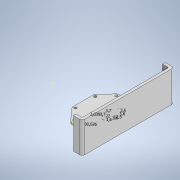
# Autodesk Inventor part: pare_choc_demo_reel
Saved by Autodesk Inventor 2020.4 (Build 244396000, 396)
## iProperties
Created: 2021-07-13
Part Number: pare_choc_demo_reel
Material: Generic
Document SubType Name: Modeling
Designer: Antonin Betaille
Density: 1 g/cm^3
Appearance: Default
Author: Antonin Betaille
Autodesk Inventor part; units mm, degrees
ref_plane "YZ Plane" through (0, 0, 0) normal (1, 0, 0) x (0, 1, 0)
ref_plane "XZ Plane" through (0, 0, 0) normal (0, 1, 0) x (-1, 0, 0)
ref_plane "XY Plane" through (0, 0, 0) normal (0, 0, 1) x (1, 0, 0)
sketch "Sketch1" plane through (0, 0, 0) normal (0, 1, 0) x (-1, 0, 0)
  line L0 (0, 34) -> (16, 16) construction
  line L1 (18.9896, 18.6575) -> (2.9896, 36.6575)
  arc A0 (2.9896, 36.6575) -> (0, 38) centre (0, 34) ccw
  arc A1 (20, 16) -> (18.9896, 18.6575) centre (16, 16) ccw
  line L2 (16, 16) -> (16, -16) construction
  line L3 (20, -16) -> (20, 16)
  line L4 (16, -16) -> (0, -34) construction
  line L5 (2.9896, -36.6575) -> (18.9896, -18.6575)
  line L6 (0, 34) -> (-44.6053, 34) construction
  line L7 (0, 38) -> (-53, 38)
  line L8 (0, -34) -> (-49, -34) construction
  line L9 (-53, -38) -> (0, -38)
  line L10 (-49, 30.0008) -> (-49, -29.9992) construction
  line L11 (-53, 38) -> (-53, -38)
  arc A2 (18.9896, -18.6575) -> (20, -16) centre (16, -16) ccw
  arc A3 (0, -38) -> (2.9896, -36.6575) centre (0, -34) ccw
  point P0 (0, 0)
  point P1 (8, 25)
  point P2 (16, 0)
  point P3 (8, -25)
  point P4 (-24.1053, 34)
  point P5 (-24.5, -34)
  point P6 (-49, 0.0008)
  dimension "d1" = 34
  dimension "d2" = 32
  dimension "d3" = 16
  dimension "d4" = 16
  dimension "d6" = 8
  dimension "d12" = 4
  dimension "d13" = 4
  dimension "d15" = 4
  dimension "d17" = 68
  dimension "d18" = 76
  dimension "d19" = 73
  dimension "d21" = 20
  dimension "d40" = 76
  dimension "d41" = 53
  constraints: 33 end point, 8 point on circle, 8 tangent, 5 midpoint, 4 centre point, 2 point on line
  measures "d1" distance of L0.start point (0, 0)
  measures "d2" distance of L2.end L0.end
  measures "d3" horizontal distance of L0.end L0.start
  measures "d4" horizontal distance of point (0, 0) L0.end
  measures "d6" diameter of A1
  measures "d12" radius of A3
  measures "d13" radius of A0
  measures "d15" radius of A2
  measures "d17" distance of L0.start L4.end
  measures "d18" distance between parallel lines of L9 L7
  measures "d19" distance between parallel lines of L11 L3
  measures "d21" distance from line of point (0, 0) L3
  measures "d40" distance of L7.end L9.start
  measures "d41" distance of L7.start L7.end
extrude "Extrusion1" add sketch "Sketch1" along normal blind 4
sketch "Sketch2" plane through (0, 4, 0) normal (0, 1, 0) x (1, 0, 0)
  line L0 (-20, 16) -> (-20, -16) projected
  point P0 (0, 0)
  point P1 (0, -34)
  point P2 (-16, 16)
  point P3 (-16, -16)
  point P4 (0, 34)
  dimension "d31" = 34
  dimension "d33" = 20
  dimension "d34" = 16
  dimension "d35" = 4
  dimension "d36" = 16
  dimension "d37" = 4
  dimension "d38" = 20
  dimension "d39" = 34
  measures "d31" distance of point (0, -34) point (0, 0)
  measures "d33" distance from line of point (0, -34) L0
  measures "d34" horizontal distance of point (0, 0) point (-16, -16)
  measures "d35" distance from line of L0 point (-16, -16)
  measures "d36" horizontal distance of point (0, 0) point (-16, 16)
  measures "d37" distance from line of L0 point (-16, 16)
  measures "d38" distance from line of L0 point (0, 34)
  measures "d39" distance of point (0, 0) point (0, 34)
hole "Hole1" at (0, 4, 34) at (-16, 4, -16) at (-16, 4, 16) at (0, 4, -34) direction (0, -1, 0) diameter 4 end through all
sketch "Sketch3" plane through (0, 4, 0) normal (0, 1, 0) x (1, 0, 0)
  line L0 (53, -70) -> (53, 70)
  line L1 (48.8, 70) -> (48.8, -70)
  line L2 (53, -38) -> (53, 38) projected
  arc A0 (53, 70) -> (48.8, 74.2) centre (48.8, 70) ccw
  arc A1 (48.8, -74.2) -> (53, -70) centre (48.8, -70) ccw
  line L3 (48.8, 74.2) -> (38.8, 74.2)
  line L4 (38.8, 74.2) -> (38.8, 70)
  line L5 (38.8, 70) -> (48.8, 70)
  line L6 (48.8, -74.2) -> (38.8, -74.2)
  line L7 (38.8, -74.2) -> (38.8, -70)
  line L8 (38.8, -70) -> (48.8, -70)
  point P0 (0, 0)
  dimension "d42" = 140
  dimension "d43" = 4.2
  dimension "d52" = 70
  dimension "d53" = 10
  dimension "d54" = 10
  constraints: 16 end point, 4 perpendicular, 4 point on circle, 4 tangent, 2 centre point, 2 coincident, 2 horizontal, 1 collinear, 1 parallel
  measures "d42" distance of L0.start L0.end
  measures "d43" distance between parallel lines of L1 L0
  measures "d52" distance from line of L5 point (0, 0)
  measures "d53" distance between parallel lines of L1 L4
  measures "d54" distance between parallel lines of L1 L7
extrude "Extrusion2" add sketch "Sketch3" along normal blind 46 and the other way blind 4
chamfer "Chamfer1" distance 2 angle 45 3 edges at (48.8, 4, 0) (48.8, 2, 38) (48.8, 2, -38)
fillet "Fillet1" radius 2 1 edges at (48.8, 25, 70)
fillet "Fillet2" radius 2 1 edges at (48.8, 25, -70)
sketch "Sketch9" plane through (0, 4, 0) normal (0, 1, 0) x (1, 0, 0)
  line L0 (21.0218, -11.6451) -> (10.117, -0.7403)
  line L1 (10.117, -0.7403) -> (10.117, 4.4923)
  line L2 (10.117, 4.4923) -> (21.0218, 15.3971)
  line L3 (21.0218, 15.3971) -> (24.6218, 13.7645)
  line L4 (24.6218, 13.7645) -> (24.6218, 11.726)
  line L5 (24.6218, 11.726) -> (28.517, 11.726)
  line L6 (28.517, 11.726) -> (32.117, 8.126)
  line L7 (32.117, 8.126) -> (32.117, -4.374)
  line L8 (32.117, -4.374) -> (28.517, -7.974)
  line L9 (28.517, -7.974) -> (24.6218, -7.974)
  line L10 (24.6218, -7.974) -> (24.6218, -10.0125)
  line L11 (24.6218, -10.0125) -> (21.0218, -11.6451)
  line L12 (28.517, -4.374) -> (24.6218, -4.374)
  line L13 (24.6218, -4.374) -> (21.8025, -7.1932)
  line L14 (21.8025, -7.1932) -> (12.7333, 1.876)
  line L15 (12.7333, 1.876) -> (21.8025, 10.9453)
  line L16 (21.8025, 10.9453) -> (24.6218, 8.126)
  line L17 (24.6218, 8.126) -> (28.517, 8.126)
  line L18 (28.517, 8.126) -> (28.517, -4.374)
  line L19 (10.117, -0.7403) -> (24.6218, 13.7645)
  line L20 (24.6218, -10.0125) -> (10.117, 4.4923)
  line L21 (21.8025, -7.1932) -> (21.8025, 10.9453)
  line L22 (21.0218, -11.6451) -> (21.0218, 15.3971)
  line L23 (24.6218, -7.974) -> (21.0218, -7.974)
  line L24 (21.8025, -7.1932) -> (21.0218, -7.974)
  line L25 (32.117, -4.374) -> (28.517, -4.374)
  line L26 (32.117, 8.126) -> (28.517, 8.126)
  line L27 (24.6218, 11.726) -> (24.6218, 8.126)
  line L28 (28.517, 8.126) -> (28.517, 11.726)
  line L29 (21.0218, -7.974) -> (24.6218, -7.974)
  line L30 (21.8025, -7.1932) -> (21.0218, -7.974)
  line L31 (21.0218, -11.6451) -> (21.0218, -7.974)
  line L32 (12.7333, 1.876) -> (10.117, -0.7403)
  line L33 (21.8025, 10.9453) -> (24.6218, 13.7645)
  line L34 (28.517, -4.374) -> (32.117, -4.374)
  line L35 (0, -38) -> (46.8, -38) projected
  point P0 (-70, 0)
  point P1 (21.0218, -6.4125)
  dimension "d467" = 3.7
  dimension "d468" = 3.7
  dimension "d469" = 12.5
  dimension "d470" = 3.6
  dimension "d471" = 3.6
  dimension "d472" = 2.0385
  dimension "d473" = 3.6
  dimension "d474" = 22
  dimension "d475" = 3.6
  dimension "d523" = 30.026
  constraints: 70 end point, 10 point on line, 8 parallel, 8 perpendicular, 4 collinear
  measures "d467" distance between parallel lines of L14 L0
  measures "d468" distance between parallel lines of L15 L2
  measures "d469" distance of L6.end L7.end
  measures "d470" horizontal distance of L7.end L8.end
  measures "d471" distance from line of L7 L5.end
  measures "d472" distance of L9.end L10.end
  measures "d473" distance between parallel lines of L7 L18
  measures "d474" distance between parallel lines of L7 L1
  measures "d475" horizontal distance of L2.end L3.end
  measures "d523" distance between parallel lines of L35 L9
extrude "Extrusion16" cut sketch "Sketch9" against normal blind 0.6 contours L22 L23 L20 L11 | L20 L23 L10 | L19 L4 L27 L16 | L25 L18 L26 L7 | L26 L28 L6
extrude "Extrusion19" cut sketch "Sketch9" against normal blind 0.3 contours L1 L20 L19 | L24 L20 L23 | L2 L22 L15 L20 | L23 L20 L13 L12 L25 L8 L9 | L3 L19 L15 L22
sketch "Sketch10" plane through (0, 4, 0) normal (0, 1, 0) x (1, 0, 0)
  line L0 (31.4873, 14.588) -> (11.8138, 14.588)
  line L1 (31.4873, 14.588) -> (31.4873, 22.6975)
  line L2 (11.8138, 22.8893) -> (11.8138, 14.588)
  line L3 (28.7873, 17.288) -> (28.7996, 22.3152)
  line L4 (28.7873, 17.288) -> (14.4873, 17.288)
  line L5 (14.4873, 17.288) -> (14.4873, 22.181)
  arc A0 (31.4873, 22.6975) -> (11.8138, 22.8893) centre (21.6443, 22.1561) ccw
  arc A1 (28.7996, 22.3152) -> (14.4873, 22.181) centre (21.6443, 22.1561) ccw
  line L6 (0, -38) -> (46.8, -38) projected
  line L7 (46.8, 38) -> (0, 38) projected
  dimension "d493" = 7.157
  dimension "d494" = 9.8579
  dimension "d495" = 2.7
  dimension "d496" = 2.6736
  dimension "d497" = 5.0272
  dimension "d498" = 19.6735
  dimension "d499" = 8.3013
  dimension "d500" = 14.3
  dimension "d520" = 19.6735
  dimension "d521" = 4.8929
  dimension "d522" = 5.986
  constraints: 12 end point, 4 point on circle, 2 centre point, 1 coincident, 1 parallel
  measures "d493" radius of A1
  measures "d494" radius of A0
  measures "d495" distance between parallel lines of L0 L4
  measures "d496" distance between parallel lines of L5 L2
  measures "d497" distance from line of L4 L3.end
  measures "d498" distance between parallel lines of L1 L2
  measures "d499" distance of L2.start L0.end
  measures "d500" distance of L3.start L4.end
  measures "d520" distance of L0.start L0.end
  measures "d521" distance of L4.end L5.end
  measures "d522" distance edge to line of A0 L7
sketch "Sketch11" plane through (0, 4, 0) normal (0, 1, 0) x (1, 0, 0)
  line L0 (16.2315, -29.314) -> (31.3715, -22.7937)
  line L1 (31.3715, -22.7937) -> (31.3715, -20.0566)
  line L2 (31.3715, -20.0566) -> (16.2315, -13.5363)
  line L3 (16.2315, -13.5363) -> (12.1356, -13.5363)
  line L4 (16.2315, -13.5363) -> (31.3715, -13.5363)
  line L5 (11.6715, -10.8363) -> (11.6715, -13.3363)
  arc A0 (12.7735, -27.8548) -> (11.6715, -29.514) centre (13.4715, -29.514) ccw
  arc A1 (11.6715, -13.3363) -> (12.773, -14.9953) centre (13.4715, -13.3363) ccw
  line L6 (12.7735, -27.8548) -> (28.0515, -21.4275)
  line L7 (12.773, -14.9953) -> (28.0515, -21.4275)
  line L8 (31.3715, -32.014) -> (11.6715, -32.014)
  line L9 (11.6715, -32.014) -> (11.6715, -29.514)
  line L10 (11.6715, -10.8363) -> (31.3715, -10.8363)
  line L11 (31.3715, -13.5363) -> (31.3715, -10.8363)
  line L12 (31.3715, -29.314) -> (16.2315, -29.314)
  line L13 (31.3715, -32.014) -> (31.3715, -29.314)
  line L14 (0, -38) -> (46.8, -38) projected
  line L15 (-20, 16) -> (-20, -16) projected
  point P0 (12.0472, -15.3794)
  dimension "d501" = 1.8
  dimension "d502" = 1.8
  dimension "d503" = 2.5
  dimension "d504" = 2.5
  dimension "d505" = 19.7
  dimension "d506" = 1.102
  dimension "d507" = 1.1016
  dimension "d509" = 15.14
  dimension "d510" = 3.32
  dimension "d511" = 2.7
  dimension "d513" = 23.3
  dimension "d514" = 23.3
  dimension "d516" = 5.986
  dimension "d517" = 19.7
  dimension "d518" = 15.14
  dimension "d519" = 31.6715
  constraints: 28 end point, 4 point on circle, 4 point on line, 4 tangent, 2 centre point, 1 parallel, 1 perpendicular
  measures "d501" radius of A0
  measures "d502" radius of A1
  measures "d503" distance of L8.end L9.end
  measures "d504" distance of L5.start L5.end
  measures "d505" distance between parallel lines of L9 L1
  measures "d506" horizontal distance of L6.start L9.end
  measures "d507" horizontal distance of L5.end L7.start
  measures "d509" distance from line of L11 L2.end
  measures "d510" distance from line of L1 L6.end
  measures "d511" distance of L4.end L10.end
  measures "d513" angle of L12 L0
  measures "d514" angle of L2 L4
  measures "d516" distance between parallel lines of L14 L8
  measures "d517" distance between parallel lines of L13 L9
  measures "d518" horizontal distance of L0.start L0.end
  measures "d519" distance between parallel lines of L15 L9
extrude "Extrusion21" cut sketch "Sketch10" against normal blind 1.2
extrude "Extrusion22" cut sketch "Sketch11" against normal blind 1.2
extrude "Extrusion23" cut sketch "Sketch9" against normal blind 0.9 contours L0 L19 L14 L22 | L27 L5 L28 L17
sketch "Sketch12" plane through (0, 2.8, 0) normal (0, 1, 0) x (1, 0, 0)
  line L0 (21.0218, -10.8363) -> (20.2129, -10.8363) projected
  line L1 (24.6218, -10.0125) -> (22.8052, -10.8363) projected
  line L2 (20.2129, -10.8363) -> (22.8052, -10.8363)
  line L3 (22.8052, -10.8363) -> (21.0218, -11.6451)
  line L4 (21.0218, -11.6451) -> (20.2129, -10.8363)
  line L5 (21.0218, -10.8363) -> (21.0218, -7.974) projected
  line L6 (21.0218, -10.8363) -> (21.0218, -11.6451)
  line L7 (21.0218, -6.4125) -> (21.0218, -7.974) projected
  line L8 (31.4873, 14.588) -> (11.8138, 14.588) projected
  line L9 (20.2127, 14.588) -> (22.8059, 14.588)
  line L10 (21.0218, 15.3971) -> (20.2127, 14.588)
  line L11 (22.8059, 14.588) -> (21.0218, 15.3971)
  line L12 (10.117, 4.4923) -> (20.2127, 14.588) projected
  line L13 (22.8059, 14.588) -> (24.6218, 13.7645) projected
  point P0 (0, 0)
  constraints: 14 end point, 4 collinear, 2 point on line, 1 horizontal
extrude "Extrusion24" add sketch "Sketch12" along normal blind 0.9 contours L8 L10 L11
extrude "Extrusion25" add sketch "Sketch12" along normal blind 0.3 contours L6 L4 L0
extrude "Extrusion26" add sketch "Sketch12" along normal blind 0.6 contours L2 L3 L6
body "Solid1"
